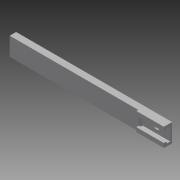
# Autodesk Inventor part: Piece Two-Diagonal Piece
Saved by Autodesk Inventor 2013 (Build 170138000, 138)
## iProperties
Created: 2014-05-23
Part Number: Piece Two-Diagonal Piece
Material: Steel
Document SubType Name: Modeling
Designer: nojessen
Density: 1 g/cm^3
Author: nojessen
Autodesk Inventor part; units mm, degrees
ref_plane "YZ Plane" through (0, 0, 0) normal (1, 0, 0) x (0, 1, 0)
ref_plane "XZ Plane" through (0, 0, 0) normal (0, 1, 0) x (-1, 0, 0)
ref_plane "XY Plane" through (0, 0, 0) normal (0, 0, 1) x (1, 0, 0)
sketch "Sketch1" plane through (0, 0, 0) normal (0, 0, 1) x (1, 0, 0)
  line L0 (0, 0) -> (215.9, 0)
  line L1 (215.9, 0) -> (215.9, 25.4)
  line L2 (215.9, 25.4) -> (0, 25.4)
  line L3 (0, 25.4) -> (0, 0)
  dimension "d0" = 215.9
  dimension "d1" = 25.4
  constraints: 8 end point, 2 parallel, 1 horizontal, 1 perpendicular
  measures "d0" distance of L2.end L1.end
  measures "d1" distance of L1.end L0.end
extrude "Extrusion1" add sketch "Sketch1" along normal blind 8.89
sketch "Sketch2" plane through (0, 0, 8.89) normal (0, 0, 1) x (1, 0, 0)
  line L0 (0, 0) -> (215.9, 0) projected
  line L1 (215.9, 25.4) -> (0, 25.4) projected
  line L2 (0, 25.4) -> (0, 0) projected
  line L3 (215.9, 25.4) -> (177.8, 25.4)
  line L4 (177.8, 25.4) -> (177.8, 0)
  line L5 (177.8, 0) -> (215.9, 0)
  line L6 (215.9, 0) -> (215.9, 25.4)
  line L7 (177.8, 0) -> (215.9, 0)
  line L8 (215.9, 0) -> (215.9, 12.7)
  line L9 (215.9, 12.7) -> (177.8, 12.7)
  line L10 (177.8, 12.7) -> (177.8, 0)
  line L11 (177.8, 12.7) -> (215.9, 12.7)
  line L12 (215.9, 12.7) -> (215.9, 3.429)
  line L13 (215.9, 3.429) -> (177.8, 3.429)
  line L14 (177.8, 3.429) -> (177.8, 12.7)
  line L15 (177.8, 12.7) -> (215.9, 12.7)
  line L16 (215.9, 12.7) -> (215.9, 21.971)
  line L17 (215.9, 21.971) -> (177.8, 21.971)
  line L18 (177.8, 21.971) -> (177.8, 12.7)
  line L19 (215.9, 25.4) -> (177.8, 25.4)
  line L20 (177.8, 25.4) -> (177.8, 21.971)
  line L21 (177.8, 21.971) -> (215.9, 21.971)
  line L22 (215.9, 21.971) -> (215.9, 25.4)
  dimension "d4" = 38.1
  dimension "d5" = 9.271
  dimension "d6" = 9.271
  constraints: 40 end point, 10 parallel, 5 horizontal, 5 perpendicular, 3 point on line, 1 midpoint
  measures "d4" distance of L5.end L4.end
  measures "d5" distance of L11.end L12.end
  measures "d6" distance of L16.end L15.end
extrude "Extrusion2" add sketch "Sketch2" along normal blind 8.89 contours L4 L13 L6 L0
sketch "Sketch3" plane through (0, 0, 8.89) normal (0, 0, 1) x (1, 0, 0)
  line L0 (215.9, 25.4) -> (177.8, 25.4)
  line L1 (177.8, 25.4) -> (177.8, 21.9726)
  line L2 (177.8, 21.9726) -> (215.9, 21.9726)
  line L3 (215.9, 21.9726) -> (215.9, 25.4)
  constraints: 8 end point, 2 parallel, 1 horizontal, 1 perpendicular
extrude "Extrusion3" add sketch "Sketch3" along normal blind 8.89
sketch "Sketch4" plane through (177.8, 3.429, 8.89) normal (0, 1, 0) x (1, 0, 0)
  line L0 (38.1, 0) -> (38.1, -8.89) projected
  line L1 (0, 0) -> (38.1, 0)
  line L2 (38.1, 0) -> (38.1, -5.08)
  line L3 (38.1, -5.08) -> (0, -5.08)
  line L4 (0, -5.08) -> (0, 0)
  line L5 (38.1, -5.08) -> (0, -5.08)
  line L6 (0, -5.08) -> (0, -8.89)
  line L7 (0, -8.89) -> (38.1, -8.89)
  line L8 (38.1, -8.89) -> (38.1, -5.08)
  point P0 (-177.8, 8.89)
  dimension "d11" = 5.08
  constraints: 16 end point, 4 parallel, 2 horizontal, 2 perpendicular, 1 point on line
  measures "d11" distance of L1.end L2.end
extrude "Extrusion4" add sketch "Sketch4" along normal blind 2.54 contours L0 L7 L6 L3
sketch "Sketch5" plane through (177.8, 21.9726, 8.89) normal (0, -1, 0) x (1, 0, 0)
  line L0 (38.1, 0) -> (38.1, 8.89) projected
  line L1 (0, 0) -> (38.1, 0)
  line L2 (38.1, 0) -> (38.1, 5.08)
  line L3 (38.1, 5.08) -> (0, 5.08)
  line L4 (0, 5.08) -> (0, 0)
  line L5 (0, 5.08) -> (38.1, 5.08)
  line L6 (38.1, 5.08) -> (38.1, 8.89)
  line L7 (38.1, 8.89) -> (0, 8.89)
  line L8 (0, 8.89) -> (0, 5.08)
  point P0 (-177.8, -8.89)
  dimension "d14" = 5.08
  constraints: 16 end point, 4 parallel, 2 horizontal, 2 perpendicular, 1 point on line
  measures "d14" distance of L2.end L1.end
extrude "Extrusion5" add sketch "Sketch5" along normal blind 2.54 contours L3 L8 L7 L0
sketch "Sketch6" plane through (215.9, 0, 0) normal (1, 0, 0) x (0, 0, -1)
  line L0 (0, 0) -> (0, 25.4) projected
  line L1 (0, 25.4) -> (-17.78, 25.4) projected
  line L2 (-13.97, 19.4326) -> (-17.78, 19.4326) projected
  line L3 (-13.97, 21.9726) -> (-13.97, 19.4326) projected
  line L4 (-13.97, 3.429) -> (-13.97, 5.969) projected
  line L5 (-17.78, 5.969) -> (-13.97, 5.969) projected
  line L6 (-8.89, 25.4) -> (-5.054, 25.4)
  line L7 (-2.54, 21.9726) -> (-7.62, 21.9726)
  line L8 (-7.62, 21.9726) -> (-7.62, 19.4326)
  line L9 (-2.54, 21.9726) -> (-2.54, 12.7008)
  line L10 (-7.62, 19.4326) -> (-11.43, 19.4326)
  line L11 (-11.43, 19.4326) -> (-11.43, 25.4)
  line L12 (-2.54, 12.7008) -> (-7.9346, 12.7008) construction
  line L13 (-2.54, 3.429) -> (-7.62, 3.429)
  line L14 (-7.62, 3.429) -> (-7.62, 5.969)
  line L15 (-2.54, 3.429) -> (-2.54, 12.7008)
  line L16 (-7.62, 5.969) -> (-11.43, 5.969)
  line L17 (-11.43, 5.969) -> (-11.43, 0.0016)
  line L18 (0, 0) -> (-17.78, 0)
  line L19 (-17.78, 0) -> (-17.78, 25.4)
  line L20 (-17.78, 25.4) -> (0, 25.4)
  line L21 (0, 25.4) -> (0, 0)
  line L22 (-8.89, 19.4326) -> (-8.89, 5.969)
  line L23 (-17.78, 5.969) -> (-13.97, 5.969)
  line L24 (-13.97, 5.969) -> (-13.97, 3.429)
  line L25 (-13.97, 3.429) -> (-11.43, 3.429)
  line L26 (-17.78, 19.4326) -> (-13.97, 19.4326)
  line L27 (-13.97, 19.4326) -> (-13.97, 21.9726)
  line L28 (-13.97, 21.9726) -> (-11.43, 21.9726)
  line L29 (-11.43, 5.969) -> (-7.62, 5.969)
  line L30 (-7.62, 5.969) -> (-7.62, 0)
  line L31 (-7.62, 0) -> (-11.43, 0)
  line L32 (-11.43, 0) -> (-11.43, 5.969)
  dimension "d19" = 3.81
  constraints: 54 end point, 6 point on line, 5 parallel, 5 symmetric about line, 4 collinear, 4 perpendicular, 3 horizontal, 1 midpoint
  measures "d19" distance of L8.end L10.end
extrude "Extrusion6" add sketch "Sketch6" against normal up to surface (38.1 mm away) contours L18 L30 L13 L15 L9 L7 L8 L10 L11 L1 L0 | L18 L17 L16 L14 L30
extrude "Extrusion7" cut sketch "Sketch6" against normal up to surface (38.1 mm away) contours L18 L19 L5 L4 L25 L17 | L14 L16 L22 L10 L8 L7 L9 L15 L13 | L25 L4 L5 L19 L2 L3 L28 L11 L10 L22 L16 L17 | L11 L28 L3 L2 L19 L1
sketch "Sketch7" plane through (0, 0, 0) normal (0, 0, -1) x (-1, 0, 0)
  line L0 (0, 0) -> (-215.9, 0) projected
  line L1 (-215.9, 25.4) -> (-177.8, 25.4)
  line L2 (-177.8, 25.4) -> (-177.8, 0)
  line L3 (-177.8, 0) -> (-215.9, 0)
  line L4 (-215.9, 0) -> (-215.9, 25.4)
  circle A0 centre (-196.85, 12.7) radius 4.445
  dimension "d24" = 38.1
  dimension "d25" = 8.89
  constraints: 8 end point, 2 parallel, 1 centre point, 1 horizontal, 1 perpendicular, 1 point on line
  measures "d24" distance of L2.end L3.end
  measures "d25" diameter of A0
extrude "Extrusion8" cut sketch "Sketch7" against normal blind 2.54 contours A0
body "Solid1"
